Autodesk Fusion 360 part; units mm, degrees
note: some values were not read from the file. Set by a fixed rule: the direction of a hole.
(part 4 of 6)
  spline S731 degree 3 poles (-127.5181, -68.7033) (-127.2038, -68.7033) (-126.8894, -68.7033) (-126.5656, -68.7033) knots 0 0 0 0 1 1 1 1
  spline S732 degree 3 poles (-126.5656, -68.7033) (-126.5656, -71.637) (-126.5656, -74.5707) (-126.5656, -77.5933) knots 0 0 0 0 1 1 1 1
  spline S733 degree 3 poles (-123.0731, -62.9883) (-123.0731, -62.7264) (-123.0731, -62.4644) (-123.0731, -62.1946) knots 0 0 0 0 1 1 1 1
  spline S734 degree 3 poles (-123.0731, -62.1946) (-122.7784, -62.0963) (-122.7784, -62.0963) (-122.4778, -61.9961) knots 0 0 0 0 1 1 1 1
  spline S735 degree 3 poles (-122.4778, -61.9961) (-121.7659, -61.727) (-121.3352, -61.4302) (-120.9973, -60.7288) knots 0 0 0 0 1 1 1 1
  spline S736 degree 3 poles (-120.9973, -60.7288) (-120.8296, -60.2267) (-120.7999, -59.8033) (-120.7849, -59.2744) knots 0 0 0 0 1 1 1 1
  spline S737 degree 3 poles (-120.7849, -59.2744) (-120.7756, -58.9882) (-120.7756, -58.9882) (-120.7663, -58.6962) knots 0 0 0 0 1 1 1 1
  spline S738 degree 3 poles (-120.7663, -58.6962) (-120.7589, -58.3995) (-120.7589, -58.3995) (-120.7514, -58.0968) knots 0 0 0 0 1 1 1 1
  spline S739 degree 3 poles (-120.7514, -58.0968) (-120.7422, -57.7956) (-120.7422, -57.7956) (-120.7328, -57.4882) knots 0 0 0 0 1 1 1 1
  spline S740 degree 3 poles (-120.7328, -57.4882) (-120.7178, -56.9933) (-120.7042, -56.4983) (-120.6918, -56.0033) knots 0 0 0 0 1 1 1 1
  spline S741 degree 3 poles (-120.6918, -56.0033) (-120.4299, -56.0033) (-120.168, -56.0033) (-119.8981, -56.0033) knots 0 0 0 0 1 1 1 1
  spline S742 degree 3 poles (-119.8981, -56.0033) (-119.8981, -58.256) (-119.8981, -60.5086) (-119.8981, -62.8296) knots 0 0 0 0 1 1 1 1
  spline S743 degree 3 poles (-119.8981, -62.8296) (-120.16, -62.8296) (-120.422, -62.8296) (-120.6918, -62.8296) knots 0 0 0 0 1 1 1 1
  spline S744 degree 3 poles (-120.6918, -62.8296) (-120.7442, -62.62) (-120.7966, -62.4105) (-120.8506, -62.1946) knots 0 0 0 0 1 1 1 1
  spline S745 degree 3 poles (-120.8506, -62.1946) (-120.975, -62.2961) (-121.0994, -62.3976) (-121.2276, -62.5021) knots 0 0 0 0 1 1 1 1
  spline S746 degree 3 poles (-121.2276, -62.5021) (-121.8807, -63.0153) (-122.2467, -63.0036) (-123.0731, -62.9883) knots 0 0 0 0 1 1 1 1
  spline S747 degree 3 poles (-70.6856, -60.2896) (-71.484, -60.1833) (-72.1646, -59.8489) (-72.8901, -59.5181) knots 0 0 0 0 1 1 1 1
  spline S748 degree 3 poles (-72.8901, -59.5181) (-73.0942, -59.4262) (-73.0942, -59.4262) (-73.3024, -59.3323) knots 0 0 0 0 1 1 1 1
  spline S749 degree 3 poles (-73.3024, -59.3323) (-73.5901, -59.2025) (-73.8777, -59.0722) (-74.165, -58.9416) knots 0 0 0 0 1 1 1 1
  spline S750 degree 3 poles (-74.165, -58.9416) (-74.6001, -58.7439) (-75.0357, -58.5474) (-75.4713, -58.3511) knots 0 0 0 0 1 1 1 1
  spline S751 degree 3 poles (-75.4713, -58.3511) (-78.1374, -57.147) (-78.1374, -57.147) (-79.4168, -56.4796) knots 0 0 0 0 1 1 1 1
  spline S752 degree 3 poles (-79.4168, -56.4796) (-79.3645, -56.27) (-79.3121, -56.0605) (-79.2581, -55.8446) knots 0 0 0 0 1 1 1 1
  spline S753 degree 3 poles (-79.2581, -55.8446) (-77.9251, -56.2478) (-76.6807, -56.8221) (-75.4183, -57.4023) knots 0 0 0 0 1 1 1 1
  spline S754 degree 3 poles (-75.4183, -57.4023) (-75.1011, -57.5475) (-74.7838, -57.6925) (-74.4664, -57.8372) knots 0 0 0 0 1 1 1 1
  spline S755 degree 3 poles (-74.4664, -57.8372) (-74.2574, -57.9325) (-74.0485, -58.0282) (-73.8397, -58.124) knots 0 0 0 0 1 1 1 1
  spline S756 degree 3 poles (-73.8397, -58.124) (-73.3173, -58.3627) (-72.7932, -58.5931) (-72.2615, -58.8102) knots 0 0 0 0 1 1 1 1
  spline S757 degree 3 poles (-72.2615, -58.8102) (-72.1586, -58.8526) (-72.0557, -58.8949) (-71.9497, -58.9386) knots 0 0 0 0 1 1 1 1
  spline S758 degree 3 poles (-71.9497, -58.9386) (-71.6668, -59.0542) (-71.3829, -59.1677) (-71.099, -59.2811) knots 0 0 0 0 1 1 1 1
  spline S759 degree 3 poles (-71.099, -59.2811) (-70.6856, -59.4958) (-70.6856, -59.4958) (-70.5268, -59.9721) knots 0 0 0 0 1 1 1 1
  spline S760 degree 3 poles (-70.5268, -59.9721) (-70.5792, -60.0768) (-70.6316, -60.1816) (-70.6856, -60.2896) knots 0 0 0 0 1 1 1 1
  spline S761 degree 3 poles (-127.5181, -62.8296) (-127.8324, -62.8296) (-128.1467, -62.8296) (-128.4706, -62.8296) knots 0 0 0 0 1 1 1 1
  spline S762 degree 3 poles (-128.4706, -62.8296) (-128.4706, -60.5769) (-128.4706, -58.3242) (-128.4706, -56.0033) knots 0 0 0 0 1 1 1 1
  spline S763 degree 3 poles (-128.4706, -56.0033) (-128.1563, -56.0033) (-127.8419, -56.0033) (-127.5181, -56.0033) knots 0 0 0 0 1 1 1 1
  spline S764 degree 3 poles (-127.5181, -56.0033) (-127.5181, -58.256) (-127.5181, -60.5086) (-127.5181, -62.8296) knots 0 0 0 0 1 1 1 1
  spline S765 degree 3 poles (-54.6518, -79.9746) (-54.9693, -79.8158) (-54.9693, -79.8158) (-55.1657, -79.2275) knots 0 0 0 0 1 1 1 1
  spline S766 degree 3 poles (-55.1657, -79.2275) (-55.2393, -78.9651) (-55.3114, -78.7023) (-55.3823, -78.4392) knots 0 0 0 0 1 1 1 1
  spline S767 degree 3 poles (-55.3823, -78.4392) (-55.4206, -78.3003) (-55.459, -78.1615) (-55.4984, -78.0184) knots 0 0 0 0 1 1 1 1
  spline S768 degree 3 poles (-55.4984, -78.0184) (-55.5794, -77.7239) (-55.6597, -77.4293) (-55.7394, -77.1344) knots 0 0 0 0 1 1 1 1
  spline S769 degree 3 poles (-55.7394, -77.1344) (-55.8613, -76.6841) (-55.9857, -76.2346) (-56.1104, -75.7851) knots 0 0 0 0 1 1 1 1
  spline S770 degree 3 poles (-56.1104, -75.7851) (-56.1886, -75.499) (-56.2668, -75.2129) (-56.3448, -74.9268) knots 0 0 0 0 1 1 1 1
  spline S771 degree 3 poles (-56.3448, -74.9268) (-56.382, -74.7925) (-56.4192, -74.6582) (-56.4575, -74.5198) knots 0 0 0 0 1 1 1 1
  spline S772 degree 3 poles (-56.4575, -74.5198) (-56.6262, -73.8905) (-56.7655, -73.3303) (-56.7156, -72.6721) knots 0 0 0 0 1 1 1 1
  spline S773 degree 3 poles (-56.7156, -72.6721) (-56.506, -72.6721) (-56.2965, -72.6721) (-56.0806, -72.6721) knots 0 0 0 0 1 1 1 1
  spline S774 degree 3 poles (-56.0806, -72.6721) (-55.5478, -74.4857) (-55.0153, -76.2996) (-54.503, -78.1192) knots 0 0 0 0 1 1 1 1
  spline S775 degree 3 poles (-54.503, -78.1192) (-54.4695, -78.2365) (-54.436, -78.3538) (-54.4015, -78.4747) knots 0 0 0 0 1 1 1 1
  spline S776 degree 3 poles (-54.4015, -78.4747) (-54.2723, -78.9375) (-54.1756, -79.3328) (-54.1756, -79.8158) knots 0 0 0 0 1 1 1 1
  spline S777 degree 3 poles (-54.1756, -79.8158) (-54.3328, -79.8682) (-54.4899, -79.9206) (-54.6518, -79.9746) knots 0 0 0 0 1 1 1 1
  spline S778 degree 3 poles (-52.7468, -50.1296) (-53.0088, -50.0772) (-53.2707, -50.0248) (-53.5406, -49.9708) knots 0 0 0 0 1 1 1 1
  spline S779 degree 3 poles (-53.5406, -49.9708) (-53.2103, -48.6991) (-52.8209, -47.4547) (-52.3996, -46.2104) knots 0 0 0 0 1 1 1 1
  spline S780 degree 3 poles (-52.3996, -46.2104) (-52.3411, -46.0366) (-52.2827, -45.8627) (-52.2225, -45.6836) knots 0 0 0 0 1 1 1 1
  spline S781 degree 3 poles (-52.2225, -45.6836) (-52.0802, -45.2605) (-51.9375, -44.8374) (-51.7943, -44.4146) knots 0 0 0 0 1 1 1 1
  spline S782 degree 3 poles (-51.7943, -44.4146) (-51.5848, -44.467) (-51.3752, -44.5193) (-51.1593, -44.5733) knots 0 0 0 0 1 1 1 1
  spline S783 degree 3 poles (-51.1593, -44.5733) (-51.2516, -45.3381) (-51.4067, -46.0337) (-51.6461, -46.7654) knots 0 0 0 0 1 1 1 1
  spline S784 degree 3 poles (-51.6461, -46.7654) (-51.7421, -47.0609) (-51.7421, -47.0609) (-51.8399, -47.3623) knots 0 0 0 0 1 1 1 1
  spline S785 degree 3 poles (-51.8399, -47.3623) (-51.9074, -47.567) (-51.9749, -47.7718) (-52.0424, -47.9765) knots 0 0 0 0 1 1 1 1
  spline S786 degree 3 poles (-52.0424, -47.9765) (-52.1106, -48.1856) (-52.1787, -48.3947) (-52.2467, -48.6038) knots 0 0 0 0 1 1 1 1
  spline S787 degree 3 poles (-52.2467, -48.6038) (-52.4126, -49.1126) (-52.5793, -49.6212) (-52.7468, -50.1296) knots 0 0 0 0 1 1 1 1
  spline S788 degree 3 poles (-127.5181, -65.6871) (-127.8324, -65.6871) (-128.1467, -65.6871) (-128.4706, -65.6871) knots 0 0 0 0 1 1 1 1
  spline S789 degree 3 poles (-128.4706, -65.6871) (-128.4706, -65.2156) (-128.4706, -64.7441) (-128.4706, -64.2583) knots 0 0 0 0 1 1 1 1
  spline S790 degree 3 poles (-128.4706, -64.2583) (-128.1563, -64.2583) (-127.8419, -64.2583) (-127.5181, -64.2583) knots 0 0 0 0 1 1 1 1
  spline S791 degree 3 poles (-127.5181, -64.2583) (-127.5181, -64.7298) (-127.5181, -65.2013) (-127.5181, -65.6871) knots 0 0 0 0 1 1 1 1
  spline S792 degree 3 poles (-126.5656, -81.0858) (-126.8799, -81.0858) (-127.1942, -81.0858) (-127.5181, -81.0858) knots 0 0 0 0 1 1 1 1
  spline S793 degree 3 poles (-127.5181, -81.0858) (-127.5181, -80.6143) (-127.5181, -80.1428) (-127.5181, -79.6571) knots 0 0 0 0 1 1 1 1
  spline S794 degree 3 poles (-127.5181, -79.6571) (-127.2038, -79.6571) (-126.8894, -79.6571) (-126.5656, -79.6571) knots 0 0 0 0 1 1 1 1
  spline S795 degree 3 poles (-126.5656, -79.6571) (-126.5656, -80.1286) (-126.5656, -80.6) (-126.5656, -81.0858) knots 0 0 0 0 1 1 1 1
extrude "Extrude4" cut sketch "Sketch2" against normal blind 0.5 contours S0 S1 S2 S3 S4 S5 S6 S7 S8 S9 S10 S11 S12 S13 S14 S15 S16 S17 S18 S19 S20 S21 S22 S23 S24 S25 S26 S27 S28 S29 S30 S31 S32 S33 S34 S35 S36 S37 S38 S39 S40 S41 S42 S43 S44 S45 S46 S47 S48 S49 S50 S51 S52 S53 S54 S55 S56 S57 S58 S59 S60 S61 S62 S63 S64 S65 S66 S67 S68 S69 S70 S71 S72 S73 S74 S75 S76 S77 S78 S79 S80 S81 S82 S83 S84 S85 S86 S87 S88 S89 S90 S91 S92 S93 S94 S95 S96 S97 S98 S99 S100 S101 S102 S103 S104 S105 S106 S107 S108 S109 S110 S111 S112 S113 S114 S115 S116 S117 S118 S119 S120 S121 S122 S123 S124 S125 S126 S127 S128 S129 S130 S131 S132 S133 S134 S135 S136 S137 S138 S139 S140 S141 S142 S143 S144 S145 S146 S147 | S148 S149 S150 S151 S152 S153 S154 S155 S156 S157 S158 S159 S160 S161 S162 S163 S164 S165 S166 S167 S168 S169 S170 S171 S172 S173 S174 S175 S176 S177 S178 S179 S180 S181 S182 S183 S184 S185 S186 S187 S188 S189 S190 S191 S192 S193 S194 S195 S196 S197 S198 S199 S200 S201 S202 S203 S204 S205 S206 S207 S208 S209 S210 S211 S212 S213 S214 S215 S216 S217 S218 S219 S220 S221 S222 S223 S224 S225 S226 S227 S228 S229 S230 S231 S232 S233 S234 S235 S236 S237 S238 | S239 S240 S241 S242 S243 S244 S245 S246 S247 S248 S249 S250 S251 S252 S253 S254 S255 S256 S257 S258 S259 S260 S261 S262 S263 S264 S265 S266 S267 | S276 S277 S278 S279 S280 S281 S282 S283 S284 S285 S286 S287 S288 S289 S290 S291 S292 S293 S294 S295 S296 S297 S298 | S308 S309 S310 S311 S312 S313 S314 S315 S316 S317 S318 S319 S320 S321 S322 | S327 S328 S329 S330 S331 S332 S333 S334 S335 S336 S337 S338 S339 S340 S341 | S346 S347 S348 S349 S350 S351 S352 S353 S354 S355 S356 S357 S358 S359 S360 S361 S362 S363 S364 S365 S366 S367 S368 S369 S370 S371 S372 S373 S374 S375 S376 S377 S378 S379 S380 S381 | S382 S383 S384 S385 S386 S387 S388 | S396 S397 S398 S399 S400 S401 S402 S403 S404 S405 S406 S407 S408 S409 S410 S411 S412 S413 S414 S415 S416 S417 S418 S419 S420 S421 S422 S423 S424 | S425 S426 S427 S428 S429 S430 S431 S432 S433 S434 S435 S436 S437 S438 S439 S440 S441 S442 S443 | S444 S445 S446 S447 S448 S449 S450 S451 S452 S453 S454 S455 S456 S457 S458 S459 S460 S461 | S462 S463 S464 S465 S466 S467 S468 S469 S470 S471 S472 S473 S474 S475 S476 S477 S478 S479 | S480 S481 S482 S483 S484 S485 S486 S487 S488 S489 S490 S491 S492 S493 S494 S495 S496 S497 S498 S499 S500 S501 S502 S503 | S504 S505 S506 S507 S508 S509 S510 | S519 S520 S521 S522 S523 S524 S525 | S533 S534 S535 S536 S537 S538 S539 S540 S541 S542 S543 S544 S545 S546 S547 S548 S549 S550 S551 S552 S553 S554 S555 S556 S557 S558 | S559 S560 S561 S562 S563 S564 S565 S566 S567 S568 S569 S570 S571 S572 S573 S574 S575 S576 S577 S578 S579 S580 S581 S582 | S583 S584 S585 S586 S587 S588 S589 S590 S591 S592 S593 S594 S595 S596 S597 S598 S599 S600 S601 S602 S603 S604 S605 S606 S607 S608 | S609 S610 S611 S612 S613 S614 S615 S616 S617 S618 S619 S620 S621 S622 S623 S624 S625 S626 S627 S628 S629 S630 S631 S632 | S633 S634 S635 S636 S637 S638 S639 S640 S641 S642 S643 S644 S645 S646 S647 S648 S649 S650 S651 S652 S653 S654 S655 | S656 S657 S658 S659 | S660 S661 S662 S663 S664 S665 S666 S667 S668 S669 S670 S671 S672 S673 S674 S675 S676 | S677 S678 S679 S680 S681 S682 S683 S684 S685 S686 S687 S688 S689 S690 S691 S692 S693 S694 S695 S696 | S697 S698 S699 S700 S701 S702 S703 S704 S705 S706 S707 S708 | S709 S710 S711 S712 S713 S714 S715 S716 S717 S718 S719 S720 S721 S722 S723 S724 S725 S726 S727 S728 | S729 S730 S731 S732 | S733 S734 S735 S736 S737 S738 S739 S740 S741 S742 S743 S744 S745 S746 | S747 S748 S749 S750 S751 S752 S753 S754 S755 S756 S757 S758 S759 S760 | S761 S762 S763 S764 | S765 S766 S767 S768 S769 S770 S771 S772 S773 S774 S775 S776 S777 | S778 S779 S780 S781 S782 S783 S784 S785 S786 S787 | S788 S789 S790 S791 | S792 S793 S794 S795 bodies 1
extrude "Extrude5" add sketch "Sketch1" along normal blind 2.5 contours L3 L7 L11 L24 L28 L29 L30 L31 | L1 L26 L32 L33 L34 L35 bodies 1
fillet "Fillet1" radius 1.5 4 edges at (15, 121, 3.75) (164, 121, 3.75) (164, 15, 3.75) (15, 15, 3.75) on bodies 1
fillet "Fillet1" radius 1.5 4 edges at (184, 136, 1.25) (-5, 136, 1.25) (184, 0, 1.25) (-5, -0.1171, 1.25) on bodies 1
equation "d3 = ( ( ( 179 - 129 ) / 2 ) * 1 ) * 1 mm - 10 mm"
equation "d4 = ( ( ( 136 - 86 ) / 2 ) * 1 ) * 1 mm - 10 mm"
equation "d5 = 15 mm + 10 mm"
equation "d6 = 15 mm + 10 mm"
equation "d7 = 129 mm + 10 mm + 10 mm"
equation "d8 = 86 mm + 10 mm + 10 mm"
equation "d11 = ( 15.5 / 2 ) * 1 mm"
equation "d12 = ( 15.5 / 2 ) * 1 mm"
equation "d14 = ( 15.75 / 2 ) * 1 mm"
equation "d16 = ( 15.75 / 2 ) * 1 mm"

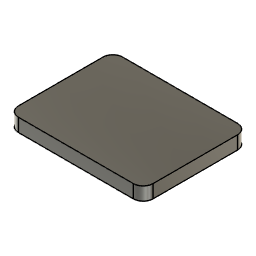
design "uv lamp"
Autodesk Fusion 360 part; units mm, degrees
sketch "Sketch1" plane through (0, 0, 0) normal (0, 0, 1) x (1, 0, 0)
  line L0 (102, -79) -> (-102, -79)
  line L1 (-102, -79) -> (-102, 79)
  line L2 (-102, 79) -> (102, 79)
  line L3 (102, 79) -> (102, -79)
  line L4 (102, -79) -> (-102, 79) construction
  line L5 (-102, -79) -> (102, 79) construction
  dimension "d1" = 204
  dimension "d2" = 158
  constraint horizontal L0
  constraint perpendicular L0 L1
  constraint parallel L0 L2
  constraint parallel L1 L3
  constraint coincident L4 origin
  constraint coincident L5 origin
  measures "d1" distance of L1.end L2.end
  measures "d2" distance of L0.end L1.end
extrude "Extrude1" add sketch "Sketch1" along normal blind 20
fillet "Fillet1" radius 15 4 edges at (102, -79, 10) (-102, -79, 10) (-102, 79, 10) (102, 79, 10)
sketch "Sketch2" plane through (0, 0, 0) normal (0, 0, -1) x (1, 0, 0)
  arc A0 (87, -79) -> (102, -64) centre (87, -64) ccw
  line L0 (102, -64) -> (102, 64)
  arc A1 (102, 64) -> (87, 79) centre (87, 64) ccw
  line L1 (87, 79) -> (-87, 79)
  arc A2 (-87, 79) -> (-102, 64) centre (-87, 64) ccw
  line L2 (-102, 64) -> (-102, -64)
  arc A3 (-102, -64) -> (-87, -79) centre (-87, -64) ccw
  line L3 (-87, -79) -> (87, -79)
  line L4 (50, -30) -> (-50, -30)
  line L5 (-50, -30) -> (-50, 30)
  line L6 (-50, 30) -> (50, 30)
  line L7 (50, 30) -> (50, -30)
  line L8 (50, -30) -> (-50, 30) construction
  line L9 (-50, -30) -> (50, 30) construction
  dimension "d7" = 100
  dimension "d8" = 60
  constraint horizontal L4
  constraint perpendicular L4 L5
  constraint parallel L4 L6
  constraint parallel L5 L7
  constraint coincident L8 origin
  constraint coincident L9 origin
  measures "d7" distance of L5.end L6.end
  measures "d8" distance of L4.end L5.end
extrude "Extrude2" add sketch "Sketch2" along normal blind 0.1 contours L4 L5 L6 L7

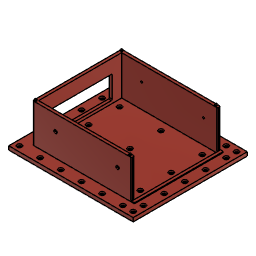
design "uv outer base"
part number: base
Autodesk Fusion 360 part; units mm, degrees
sketch "Sketch1" plane through (0, 0, 0) normal (0, 0, 1) x (1, 0, 0)
  line L0 (0, 0) -> (232, 0)
  line L1 (232, 0) -> (232, 201)
  line L2 (232, 201) -> (0, 201)
  line L3 (0, 201) -> (0, 0)
  line L4 (0, 201) -> (-7, 201)
  line L5 (0, 201) -> (-7, 201)
  line L6 (-7, 201) -> (-7, 208)
  line L7 (-7, 208) -> (0, 208)
  line L8 (0, 208) -> (0, 201)
  line L9 (232, 0) -> (239, 0)
  line L10 (239, 0) -> (239, -7)
  line L11 (239, -7) -> (232, -7)
  line L12 (232, -7) -> (232, 0)
  line L13 (-7, 208) -> (239, 208)
  line L14 (239, 208) -> (239, -7)
  line L15 (239, -7) -> (-7, -7)
  line L16 (-7, -7) -> (-7, 208)
  line L17 (232, 201) -> (232, 208)
  line L18 (239, 208) -> (239, 240.3287)
  line L19 (-21.5407, 238.3287) -> (-21.5407, 225.3287)
  line L20 (-21.5407, 225.3287) -> (-34.5407, 225.3287)
  circle A0 centre (-21.5407, -24.6713) radius 5.75
  line L21 (266.4593, -37.6713) -> (253.4593, -37.6713)
  circle A1 centre (-21.5407, 25.3287) radius 3
  line L22 (253.4593, -37.6713) -> (253.4593, -24.6713)
  circle A2 centre (-21.5407, 225.3287) radius 5.75
  line L23 (-34.5407, 238.3287) -> (-21.5407, 238.3287)
  line L24 (-34.5407, 225.3287) -> (-34.5407, 238.3287)
  line L25 (253.4593, -24.6713) -> (266.4593, -24.6713)
  circle A3 centre (28.4593, -24.6713) radius 3
  circle A4 centre (-21.5407, 225.3287) radius 3
  circle A5 centre (253.4593, 0.3287) radius 5.75
  line L26 (266.4593, -24.6713) -> (266.4593, -37.6713)
  circle A6 centre (253.4593, -24.6713) radius 5.75
  circle A7 centre (-21.5407, 25.3287) radius 5.75
  circle A8 centre (253.4593, -24.6713) radius 3
  circle A9 centre (-21.5407, 75.3287) radius 3
  circle A10 centre (253.4593, 0.3287) radius 3
  circle A11 centre (253.4593, 50.3287) radius 5.75
  circle A12 centre (253.4593, 50.3287) radius 3
  circle A13 centre (128.4593, -24.6713) radius 5.75
  circle A14 centre (78.4593, -24.6713) radius 3
  circle A15 centre (28.4593, 225.3287) radius 3
  circle A16 centre (-21.5407, -24.6713) radius 3
  circle A17 centre (228.4593, -24.6713) radius 3
  circle A18 centre (78.4593, -24.6713) radius 5.75
  circle A19 centre (253.4593, 225.3287) radius 3
  circle A20 centre (253.4593, 225.3287) radius 5.75
  circle A21 centre (-21.5407, 175.3287) radius 3
  circle A22 centre (-21.5407, 125.3287) radius 3
  circle A23 centre (-21.5407, 125.3287) radius 5.75
  circle A24 centre (28.4593, -24.6713) radius 5.75
  circle A25 centre (-21.5407, 175.3287) radius 5.75
  line L27 (232.8, 201) -> (232.8, 208)
  circle A26 centre (78.4593, 225.3287) radius 3
  circle A27 centre (178.4593, 225.3287) radius 5.75
  circle A28 centre (128.4593, 225.3287) radius 5.75
  circle A29 centre (178.4593, 225.3287) radius 3
  circle A30 centre (178.4593, -24.6713) radius 3
  circle A31 centre (128.4593, -24.6713) radius 3
  circle A32 centre (28.4593, 225.3287) radius 5.75
  circle A33 centre (228.4593, 225.3287) radius 5.75
  circle A34 centre (253.4593, 200.3287) radius 3
  line L28 (266.4593, 238.3287) -> (266.4593, -37.6713)
  circle A35 centre (128.4593, 225.3287) radius 3
  circle A36 centre (-21.5407, 75.3287) radius 5.75
  circle A37 centre (228.4593, 225.3287) radius 3
  line L29 (266.4593, -37.6713) -> (-34.5407, -37.6713)
  line L30 (-34.5407, -37.6713) -> (-34.5407, 238.3287)
  circle A38 centre (228.4593, -24.6713) radius 5.75
  circle A39 centre (78.4593, 225.3287) radius 5.75
  circle A40 centre (178.4593, -24.6713) radius 5.75
  circle A41 centre (253.4593, 200.3287) radius 5.75
  line L31 (-34.5407, 238.3287) -> (266.4593, 238.3287)
  circle A42 centre (253.4593, 100.3287) radius 5.75
  circle A43 centre (253.4593, 150.3287) radius 3
  circle A44 centre (253.4593, 100.3287) radius 3
  circle A45 centre (253.4593, 150.3287) radius 5.75
  circle A46 centre (16, 180) radius 3.375
  circle A47 centre (16, 180) radius 5.75
  circle A48 centre (116, 180) radius 3.375
  circle A49 centre (116, 180) radius 5.75
  circle A50 centre (216, 180) radius 3.375
  circle A51 centre (216, 180) radius 5.75
  circle A52 centre (16, 105) radius 3.375
  circle A53 centre (16, 105) radius 5.75
  circle A54 centre (116, 105) radius 3.375
  circle A55 centre (116, 105) radius 5.75
  circle A56 centre (216, 105) radius 3.375
  circle A57 centre (216, 105) radius 5.75
  circle A58 centre (16, 30) radius 3.375
  circle A59 centre (16, 30) radius 5.75
  circle A60 centre (116, 30) radius 3.375
  circle A61 centre (116, 30) radius 5.75
  circle A62 centre (216, 30) radius 3.375
  circle A63 centre (216, 30) radius 5.75
  point P0 (0.8, 0)
  point P1 (0.8, 0)
  point P2 (0.8, 0)
  dimension "d2" = 201
  dimension "d3" = 7
  dimension "d4" = 7
  dimension "d5" = 7
  dimension "d6" = 7
  dimension "d56" = 7
  dimension "d156" = 25
  dimension "d157" = -25
  dimension "d160" = 25
  dimension "d161" = -25
  dimension "d162" = 11.5
  dimension "d163" = 6
  dimension "d164" = 13
  dimension "d165" = 13
  dimension "d166" = 13
  dimension "d167" = 13
  dimension "d168" = 7
  dimension "d223" = 6.75
  dimension "d224" = 11.5
  dimension "d227" = 100
  dimension "d228" = -75
  constraint vertical L1
  constraint horizontal L2
  constraint vertical L3
  constraint coincident L0.start L3.end
  constraint perpendicular L3 L4
  constraint horizontal L5
  constraint vertical L6
  constraint horizontal L7
  constraint vertical L8
  constraint horizontal L13
  constraint vertical L14
  constraint vertical L16
  constraint perpendicular L13 L17
  constraint concentric A2 A4
  constraint horizontal L20
  constraint vertical L24
  constraint horizontal L23
  constraint vertical L19
  constraint coincident L19.end L20.start
  constraint horizontal L25
  constraint vertical L26
  constraint horizontal L21
  constraint vertical L22
  constraint coincident L22.end L25.start
  constraint horizontal L29
  constraint vertical L30
  constraint horizontal L31
  constraint vertical L28
  constraint concentric A46 A47
  measures "d2" distance of L0.start L2.end
  measures "d3" distance of L2.end L4.end
  measures "d4" distance of L2.end L4.end
  measures "d5" distance of L2.end L7.end
  measures "d6" distance of L0.end L9.end
  measures "d56" distance of L1.end L17.end
  measures "d162" diameter of A2
  measures "d163" diameter of A4
  measures "d164" distance of L19.end L20.end
  measures "d165" distance of L19.end L19.start
  measures "d166" distance of L22.end L25.end
  measures "d167" distance of L22.end L21.end
  measures "d168" distance of L27.end L27.start
  measures "d223" diameter of A46
  measures "d224" diameter of A47
sketch "Sketch2" plane through (0, 0, 0) normal (0, 0, 1) x (1, 0, 0)
  circle A0 centre (-22.3407, 225.3287) radius 5.75
  circle A1 centre (27.6593, 225.3287) radius 5.75
  circle A2 centre (77.6593, 225.3287) radius 5.75
  circle A3 centre (127.6593, 225.3287) radius 5.75
  circle A4 centre (177.6593, 225.3287) radius 5.75
  circle A5 centre (227.6593, 225.3287) radius 5.75
  circle A6 centre (252.6593, 225.3287) radius 5.75
  circle A7 centre (252.6593, 200.3287) radius 5.75
  circle A8 centre (-22.3407, 175.3287) radius 5.75
  circle A9 centre (252.6593, 150.3287) radius 5.75
  circle A10 centre (-22.3407, 125.3287) radius 5.75
  circle A11 centre (252.6593, 100.3287) radius 5.75
  circle A12 centre (-22.3407, 75.3287) radius 5.75
  circle A13 centre (252.6593, 50.3287) radius 5.75
  circle A14 centre (-22.3407, 25.3287) radius 5.75
  circle A15 centre (252.6593, 0.3287) radius 5.75
  circle A16 centre (-22.3407, -24.6713) radius 5.75
  circle A17 centre (27.6593, -24.6713) radius 5.75
  circle A18 centre (77.6593, -24.6713) radius 5.75
  circle A19 centre (127.6593, -24.6713) radius 5.75
  circle A20 centre (177.6593, -24.6713) radius 5.75
  circle A21 centre (227.6593, -24.6713) radius 5.75
  circle A22 centre (252.6593, -24.6713) radius 5.75
  circle A23 centre (-22.3407, 225.3287) radius 3
  circle A24 centre (27.6593, 225.3287) radius 3
  circle A25 centre (77.6593, 225.3287) radius 3
  circle A26 centre (127.6593, 225.3287) radius 3
  circle A27 centre (177.6593, 225.3287) radius 3
  circle A28 centre (227.6593, 225.3287) radius 3
  circle A29 centre (252.6593, 225.3287) radius 3
  circle A30 centre (252.6593, 200.3287) radius 3
  circle A31 centre (-22.3407, 175.3287) radius 3
  circle A32 centre (252.6593, 150.3287) radius 3
  circle A33 centre (-22.3407, 125.3287) radius 3
  circle A34 centre (252.6593, 100.3287) radius 3
  circle A35 centre (-22.3407, 75.3287) radius 3
  circle A36 centre (252.6593, 50.3287) radius 3
  circle A37 centre (-22.3407, 25.3287) radius 3
  circle A38 centre (252.6593, 0.3287) radius 3
  circle A39 centre (-22.3407, -24.6713) radius 3
  circle A40 centre (27.6593, -24.6713) radius 3
  circle A41 centre (77.6593, -24.6713) radius 3
  circle A42 centre (127.6593, -24.6713) radius 3
  circle A43 centre (177.6593, -24.6713) radius 3
  circle A44 centre (227.6593, -24.6713) radius 3
  circle A45 centre (252.6593, -24.6713) radius 3
  line L0 (-22.3407, 225.3287) -> (-35.3407, 225.3287)
  line L1 (-35.3407, 225.3287) -> (-35.3407, 238.3287)
  line L2 (-35.3407, 238.3287) -> (-22.3407, 238.3287)
  line L3 (-22.3407, 238.3287) -> (-22.3407, 225.3287)
  line L4 (252.6593, -24.6713) -> (265.6593, -24.6713)
  line L5 (265.6593, -24.6713) -> (265.6593, -37.6713)
  line L6 (265.6593, -37.6713) -> (252.6593, -37.6713)
  line L7 (252.6593, -37.6713) -> (252.6593, -24.6713)
  line L8 (265.6593, -37.6713) -> (-35.3407, -37.6713)
  line L9 (-35.3407, -37.6713) -> (-35.3407, 238.3287)
  line L10 (-35.3407, 238.3287) -> (265.6593, 238.3287)
  line L11 (265.6593, 238.3287) -> (265.6593, -37.6713)
  line L12 (232, 201) -> (232, 208)
  dimension "d8" = 11.5
  dimension "d11" = 25
  dimension "d12" = -25
  dimension "d13" = 6
  dimension "d16" = 25
  dimension "d17" = -25
  dimension "d18" = 13
  dimension "d19" = 13
  dimension "d20" = 13
  dimension "d21" = 13
  dimension "d153" = 7
  constraint concentric A0 A23
  constraint horizontal L0
  constraint vertical L1
  constraint horizontal L2
  constraint vertical L3
  constraint coincident A0.centre A23.centre
  constraint horizontal L4
  constraint vertical L5
  constraint horizontal L6
  constraint vertical L7
  constraint coincident A22.centre A45.centre
  constraint horizontal L8
  constraint vertical L9
  constraint horizontal L10
  constraint vertical L11
  measures "d8" diameter of A0
  measures "d13" diameter of A23
  measures "d18" distance of A0.centre L0.end
  measures "d19" distance of A0.centre L2.end
  measures "d20" distance of A22.centre L4.end
  measures "d21" distance of A22.centre L6.end
  measures "d153" distance of L12.start L12.end
extrude "Extrude3" add sketch "Sketch1" along normal blind 7 contours L0 L1 L2 L3 | L0 L3 L4 L5 L12 L15 L16 | L1 L9 L13 L14 L17 | L9 L10 L11 L12 L14 L15 | L2 L8 L13 L17 | L4 L5 L6 L7 L8 L13 L16 makes body 1
extrude "Extrude4" add sketch "Sketch1" along normal blind 102 contours L0 L3 L4 L5 L12 L15 L16 | L2 L8 L13 L17 | L4 L5 L6 L7 L8 L13 L16 bodies 1
sketch "Sketch4" plane through (0, 0, 102) normal (0, 0, 1) x (-1, 0, 0)
  line L0 (0, -201) -> (-232, -201)
  line L1 (-232, -201) -> (-232, -208)
  line L2 (-232, -208) -> (7, -208)
  line L3 (7, -208) -> (7, 7)
  line L4 (7, 7) -> (-232, 7)
  line L5 (-232, 0) -> (0, 0)
  line L6 (0, 0) -> (0, -201)
  line L7 (7, -208) -> (-232, -208)
  line L8 (-232, -208) -> (-232, 0)
  line L9 (-232, 0) -> (7, 0)
  line L10 (7, 0) -> (7, -208)
  line L11 (-36, -158) -> (-198, -158)
  line L12 (-198, -158) -> (-198, -43)
  line L13 (-198, -43) -> (-36, -43)
  line L14 (-36, -43) -> (-36, -158)
  line L15 (7, -208) -> (-232, -208)
  line L16 (-232, -208) -> (-232, 7)
  line L17 (-232, 7) -> (7, 7)
  line L18 (7, 7) -> (7, -208)
  line L19 (-232, 7) -> (-225, 7)
  line L20 (-225, 7) -> (-225, 3.5)
  line L21 (-225, 3.5) -> (-232, 3.5)
  line L22 (-232, 3.5) -> (-232, 7)
  line L23 (7, 7) -> (3.5, 7)
  line L24 (3.5, 7) -> (3.5, 3.5)
  line L25 (3.5, 3.5) -> (7, 3.5)
  line L26 (7, 3.5) -> (7, 7)
  line L27 (7, -208) -> (3.5, -208)
  line L28 (3.5, -208) -> (3.5, -204.5)
  line L29 (3.5, -204.5) -> (7, -204.5)
  line L30 (7, -204.5) -> (7, -208)
  line L31 (-232, -208) -> (-225, -208)
  line L32 (-225, -208) -> (-225, -204.5)
  line L33 (-225, -204.5) -> (-232, -204.5)
  line L34 (-232, -204.5) -> (-232, -208)
  line L35 (1.625, -202.625) -> (5.375, -202.625)
  line L36 (5.375, -202.625) -> (5.375, -206.375)
  line L37 (5.375, -206.375) -> (1.625, -206.375)
  line L38 (1.625, -206.375) -> (1.625, -202.625)
  line L39 (1.625, -202.625) -> (5.375, -206.375) construction
  line L40 (5.375, -202.625) -> (1.625, -206.375) construction
  line L41 (1.625, 5.375) -> (5.375, 5.375)
  line L42 (5.375, 5.375) -> (5.375, 1.625)
  line L43 (5.375, 1.625) -> (1.625, 1.625)
  line L44 (1.625, 1.625) -> (1.625, 5.375)
  line L45 (1.625, 5.375) -> (5.375, 1.625) construction
  line L46 (5.375, 5.375) -> (1.625, 1.625) construction
  line L47 (-226.875, 5.375) -> (-223.125, 5.375)
  line L48 (-223.125, 5.375) -> (-223.125, 1.625)
  line L49 (-223.125, 1.625) -> (-226.875, 1.625)
  line L50 (-226.875, 1.625) -> (-226.875, 5.375)
  line L51 (-226.875, 5.375) -> (-223.125, 1.625) construction
  line L52 (-223.125, 5.375) -> (-226.875, 1.625) construction
  line L53 (-226.875, -202.625) -> (-223.125, -202.625)
  line L54 (-223.125, -202.625) -> (-223.125, -206.375)
  line L55 (-223.125, -206.375) -> (-226.875, -206.375)
  line L56 (-226.875, -206.375) -> (-226.875, -202.625)
  line L57 (-226.875, -202.625) -> (-223.125, -206.375) construction
  line L58 (-223.125, -202.625) -> (-226.875, -206.375) construction
  line L59 (-36, -158) -> (-15.2, -158)
  line L60 (-15.2, -158) -> (-15.2, -179.35)
  line L61 (-15.2, -179.35) -> (-36, -179.35)
  line L62 (-36, -179.35) -> (-36, -158)
  line L63 (-198, -43) -> (-218.8, -43)
  line L64 (-218.8, -43) -> (-218.8, -21.65)
  line L65 (-218.8, -21.65) -> (-198, -21.65)
  line L66 (-198, -21.65) -> (-198, -43)
  line L67 (-15.2, -179.35) -> (-218.8, -179.35)
  line L68 (-218.8, -179.35) -> (-218.8, -21.65)
  line L69 (-218.8, -21.65) -> (-15.2, -21.65)
  line L70 (-15.2, -21.65) -> (-15.2, -179.35)
  line L71 (-15.2, -179.35) -> (-10.2, -179.35)
  line L72 (-10.2, -179.35) -> (-10.2, -184.35)
  line L73 (-10.2, -184.35) -> (-15.2, -184.35)
  line L74 (-15.2, -184.35) -> (-15.2, -179.35)
  line L75 (-218.8, -21.65) -> (-223.8, -21.65)
  line L76 (-223.8, -21.65) -> (-223.8, -16.65)
  line L77 (-223.8, -16.65) -> (-218.8, -16.65)
  line L78 (-218.8, -16.65) -> (-218.8, -21.65)
  line L79 (-10.2, -184.35) -> (-223.8, -184.35)
  line L80 (-223.8, -184.35) -> (-223.8, -16.65)
  line L81 (-223.8, -16.65) -> (-10.2, -16.65)
  line L82 (-10.2, -16.65) -> (-10.2, -184.35)
  line L83 (-232, 7) -> (-232, 0)
  point P0 (3.5, -204.5)
  point P1 (3.5, 3.5)
  point P2 (-225, 3.5)
  point P3 (-225, -204.5)
  dimension "d59" = 162
  dimension "d60" = 115
  dimension "d89" = 7
  dimension "d90" = 3.5
  dimension "d91" = 3.5
  dimension "d92" = 3.5
  dimension "d93" = 3.5
  dimension "d94" = 3.5
  dimension "d95" = 7
  dimension "d96" = 3.75
  dimension "d97" = 3.75
  dimension "d98" = 3.75
  dimension "d99" = 3.75
  dimension "d100" = 3.75
  dimension "d101" = 3.75
  dimension "d102" = 3.75
  dimension "d103" = 3.75
  dimension "d104" = 20.8
  dimension "d105" = 21.35
  dimension "d106" = 20.8
  dimension "d107" = 21.35
  dimension "d108" = 5
  dimension "d109" = 5
  dimension "d110" = 5
  dimension "d111" = 5
  dimension "d112" = 3.5
  constraint horizontal L7
  constraint vertical L8
  constraint horizontal L9
  constraint vertical L10
  constraint coincident L5.start L8.end
  constraint coincident L2.end L3.start
  constraint horizontal L11
  constraint vertical L12
  constraint horizontal L13
  constraint vertical L14
  constraint horizontal L15
  constraint vertical L16
  constraint horizontal L17
  constraint vertical L18
  constraint coincident L4.end L16.end
  constraint horizontal L19
  constraint vertical L20
  constraint horizontal L21
  constraint vertical L22
  constraint horizontal L23
  constraint vertical L24
  constraint horizontal L25
  constraint vertical L26
  constraint coincident L3.end L4.start
  constraint horizontal L27
  constraint vertical L28
  constraint horizontal L29
  constraint vertical L30
  constraint horizontal L31
  constraint vertical L32
  constraint horizontal L33
  constraint vertical L34
  constraint horizontal L35
  constraint perpendicular L35 L36
  constraint parallel L35 L37
  constraint parallel L36 L38
  constraint coincident L39 P0
  constraint coincident L40 P0
  constraint coincident P0 L28.end
  constraint horizontal L41
  constraint perpendicular L41 L42
  constraint parallel L41 L43
  constraint parallel L42 L44
  constraint coincident L45 P1
  constraint coincident L46 P1
  constraint coincident P1 L24.end
  constraint horizontal L47
  constraint perpendicular L47 L48
  constraint parallel L47 L49
  constraint parallel L48 L50
  constraint coincident L51 P2
  constraint coincident L52 P2
  constraint coincident P2 L20.end
  constraint horizontal L53
  constraint perpendicular L53 L54
  constraint parallel L53 L55
  constraint parallel L54 L56
  constraint coincident L57 P3
  constraint coincident L58 P3
  constraint coincident P3 L32.end
  constraint horizontal L59
  constraint vertical L60
  constraint horizontal L61
  constraint vertical L62
  constraint horizontal L63
  constraint vertical L64
  constraint horizontal L65
  constraint vertical L66
  constraint horizontal L67
  constraint vertical L68
  constraint horizontal L69
  constraint vertical L70
  constraint horizontal L71
  constraint vertical L72
  constraint horizontal L73
  constraint vertical L74
  constraint horizontal L75
  constraint vertical L76
  constraint horizontal L77
  constraint vertical L78
  constraint horizontal L79
  constraint vertical L80
  constraint horizontal L81
  constraint vertical L82
  measures "d59" distance of L11.start L11.end
  measures "d60" distance of L11.start L13.end
  measures "d89" distance of L4.end L19.end
  measures "d90" distance of L4.end L21.end
  measures "d91" distance of L3.end L23.end
  measures "d92" distance of L3.end L25.end
  measures "d93" distance of L2.end L27.end
  measures "d94" distance of L2.end L29.end
  measures "d95" distance of L1.end L31.end
  measures "d96" distance of L36.end L37.end
  measures "d97" distance of L35.end L36.end
  measures "d98" distance of L42.end L43.end
  measures "d99" distance of L41.end L42.end
  measures "d100" distance of L48.end L49.end
  measures "d101" distance of L47.end L48.end
  measures "d102" distance of L54.end L55.end
  measures "d103" distance of L53.end L54.end
  measures "d104" distance of L11.start L59.end
  measures "d105" distance of L11.start L61.end
  measures "d106" distance of L12.end L63.end
  measures "d107" distance of L12.end L65.end
  measures "d108" distance of L60.end L71.end
  measures "d109" distance of L60.end L73.end
  measures "d110" distance of L64.end L75.end
  measures "d111" distance of L64.end L77.end
  measures "d112" distance of L1.end L33.end
extrude "Extrude5" add sketch "Sketch1" along normal blind 11 contours L1 L9 L13 L14 L17 | L9 L10 L11 L12 L14 L15 bodies 1
sketch "Sketch5" plane through (0, -7, 0) normal (0, -1, 0) x (1, 0, 0)
  line L0 (-7, 0) -> (239, 0)
  line L1 (232, 11) -> (232, 102)
  line L2 (-7, 102) -> (-7, 0)
  line L3 (-7, 102) -> (15, 102)
  line L4 (0, 0) -> (0, 7)
  line L5 (15, 102) -> (232, 102)
  line L6 (232, 102) -> (232, 5.2162)
  line L7 (232, 5.2162) -> (15, 5.2162)
  line L8 (15, 5.2162) -> (15, 102)
  line L9 (0, 7) -> (48, 7)
  line L10 (48, 7) -> (48, 64.5)
  line L11 (48, 64.5) -> (0, 64.5)
  line L12 (0, 64.5) -> (0, 7)
  line L13 (48, 64.5) -> (198, 64.5)
  circle A0 centre (48, 64.5) radius 2.25
  circle A1 centre (198, 64.5) radius 2.25
  circle A2 centre (48, 64.5) radius 4
  circle A3 centre (198, 64.5) radius 4
  line L14 (232, 102) -> (-7, 102)
  line L15 (-7, 0) -> (-7, 5)
  line L16 (239, 0) -> (239, 11)
  line L17 (239, 11) -> (232, 11)
  dimension "d65" = 22
  dimension "d66" = 7
  dimension "d67" = 48
  dimension "d68" = 57.5
  dimension "d69" = 150
  dimension "d70" = 4.5
  dimension "d71" = 4.5
  dimension "d81" = 8
  dimension "d82" = 8
  constraint coincident L2.start L3.start
  constraint perpendicular L2 L3
  constraint coincident L4.start origin
  constraint perpendicular L0 L4
  constraint horizontal L5
  constraint vertical L6
  constraint horizontal L7
  constraint vertical L8
  constraint coincident L1 L6.end
  constraint horizontal L9
  constraint vertical L10
  constraint horizontal L11
  constraint vertical L12
  constraint perpendicular L10 L13
  constraint coincident L10.end L11.start
  constraint coincident L13.end A1.centre
  constraint concentric A0 A2
  constraint concentric A1 A3
  constraint coincident L0.start L2.end
  constraint coincident L2 L15.end
  constraint perpendicular L0 L15
  measures "d65" distance of L2.start L3.end
  measures "d66" distance of L4.start L4.end
  measures "d67" distance of L4.end L9.end
  measures "d68" distance of L4.end L11.end
  measures "d69" distance of L10.end L13.end
  measures "d70" diameter of A0
  measures "d71" diameter of A1
  measures "d81" diameter of A2
  measures "d82" diameter of A3
sketch "Sketch6" plane through (0, 208, 0) normal (0, 1, 0) x (-1, 0, 0)
  line L0 (-239, 0) -> (7, 0)
  line L1 (7, 0) -> (7, 102)
  line L2 (-232, 102) -> (-232, 11)
  line L3 (7, 0) -> (-15, 0)
  line L4 (-15, 0) -> (-15, 7)
  line L5 (-15, 7) -> (7, 7)
  line L6 (7, 7) -> (7, 0)
  line L7 (-15, 7) -> (-48, 7)
  line L8 (-48, 7) -> (-48, 64.5)
  line L9 (-48, 64.5) -> (-15, 64.5)
  line L10 (-15, 64.5) -> (-15, 7)
  line L11 (-48, 64.5) -> (-198, 64.5)
  circle A0 centre (-198, 64.5) radius 2.25
  circle A1 centre (-48, 64.5) radius 2.25
  circle A2 centre (-198, 64.5) radius 4
  circle A3 centre (-48, 64.5) radius 4
  line L12 (7, 102) -> (-232, 102)
  line L13 (-232, 11) -> (-239, 11)
  line L14 (-239, 11) -> (-239, 0)
  dimension "d72" = 22
  dimension "d73" = 7
  dimension "d74" = 33
  dimension "d75" = 57.5
  dimension "d76" = 150
  dimension "d77" = 4.5
  dimension "d78" = 4.5
  dimension "d83" = 8
  dimension "d84" = 8
  constraint horizontal L3
  constraint vertical L4
  constraint horizontal L5
  constraint vertical L6
  constraint coincident L0.end L1.start
  constraint horizontal L7
  constraint vertical L8
  constraint horizontal L9
  constraint vertical L10
  constraint horizontal L11
  constraint coincident L11.end A0.centre
  constraint coincident L8.end L9.start
  constraint concentric A0 A2
  constraint concentric A1 A3
  measures "d72" distance of L0.end L3.end
  measures "d73" distance of L0.end L5.end
  measures "d74" distance of L4.end L7.end
  measures "d75" distance of L4.end L9.end
  measures "d76" distance of L8.end L11.end
  measures "d77" diameter of A0
  measures "d78" diameter of A1
  measures "d83" diameter of A2
  measures "d84" diameter of A3
extrude "Extrude7" cut sketch "Sketch5" against normal blind 221 contours L11 L13 A0 | L10 L11 A0 | L10 L13 A0 | A1 bodies 1
extrude "Extrude8" cut sketch "Sketch6" against normal blind 3 contours L8 L11 A1 A3 | L8 L9 A1 A3 | L9 L11 A1 A3 | A2 bodies 1
extrude "Extrude9" cut sketch "Sketch5" against normal blind 3 contours L11 L13 A0 A2 | L10 L11 A0 A2 | L10 L13 A0 A2 | A3 bodies 1
sketch "Sketch7" plane through (0, 0, 0) normal (0, 0, 1) x (1, 0, 0)
  line L0 (632.0908, 17.9092) -> (400, 17.9092)
  line L1 (398.5, -2.5) -> (398.5, -6.5)
  line L2 (398.5, 201.5) -> (394.5, 205.5) construction
  line L3 (422.9, 178.85) -> (417.9, 178.85)
  line L4 (422.9, 183.85) -> (422.9, 178.85)
  line L5 (393, -8) -> (393, 207)
  line L6 (393, -8) -> (632, -8)
  line L7 (393, 207) -> (393, -8)
  line L8 (396.5, 207) -> (396.5, 203.5)
  line L9 (400, 17.9092) -> (400, 200)
  line L10 (393, -4.5) -> (393, -8)
  line L11 (632, 207) -> (393, 207)
  line L12 (398.5, 205.5) -> (398.5, 201.5)
  line L13 (393, 203.5) -> (393, 207)
  line L14 (632, 200) -> (632, 207)
  line L15 (394.5, 201.5) -> (394.5, 205.5)
  line L16 (396.5, -8) -> (396.5, -4.5)
  line L17 (417.9, 178.85) -> (417.9, 183.85)
  line L18 (632, -8) -> (632.0908, 17.9092)
  line L19 (394.5, -6.5) -> (398.5, -2.5) construction
  line L20 (394.5, -6.5) -> (394.5, -2.5)
  line L21 (394.5, 201.5) -> (398.5, 205.5) construction
  line L22 (400, 200) -> (632, 200)
  line L23 (396.5, -4.5) -> (393, -4.5)
  line L24 (393, 207) -> (632, 207)
  line L25 (625, 207) -> (625, 203.5)
  line L26 (627, -6.5) -> (623, -2.5) construction
  line L27 (623, -6.5) -> (623, -2.5)
  line L28 (632, 207) -> (625, 207)
  line L29 (623, -6.5) -> (627, -2.5) construction
  line L30 (623, 201.5) -> (627, 205.5) construction
  line L31 (632, 207) -> (632, -8)
  line L32 (625, -4.5) -> (632, -4.5)
  line L33 (623, -2.5) -> (627, -2.5)
  line L34 (627, -6.5) -> (623, -6.5)
  line L35 (627, -2.5) -> (627, -6.5)
  line L36 (627, 201.5) -> (623, 205.5) construction
  line L37 (632, -4.5) -> (632, -8)
  line L38 (398.5, -6.5) -> (394.5, -2.5) construction
  line L39 (393, 207) -> (396.5, 207)
  line L40 (398.5, -6.5) -> (394.5, -6.5)
  line L41 (394.5, 205.5) -> (398.5, 205.5)
  line L42 (417.9, 183.85) -> (422.9, 183.85)
  line L43 (394.5, -2.5) -> (398.5, -2.5)
  line L44 (632, -8) -> (393, -8)
  line L45 (393, -1) -> (393, 207)
  line L46 (393, -8) -> (396.5, -8)
  line L47 (632.0908, 17.9092) -> (393, -1)
  line L48 (627, 205.5) -> (627, 201.5)
  line L49 (632, 203.5) -> (632, 207)
  line L50 (631.5, 16.15) -> (626.5, 16.15)
  line L51 (632, -8) -> (625, -8)
  line L52 (625, 203.5) -> (632, 203.5)
  line L53 (625, -8) -> (625, -4.5)
  line L54 (398.5, 201.5) -> (394.5, 201.5)
  line L55 (631.5, 21.15) -> (631.5, 16.15)
  line L56 (632, 207) -> (632.0908, 17.9092)
  line L57 (393, 207) -> (632, 207)
  line L58 (623, 201.5) -> (623, 205.5)
  line L59 (623, 205.5) -> (627, 205.5)
  line L60 (627, 201.5) -> (623, 201.5)
  line L61 (396.5, 203.5) -> (393, 203.5)
  line L62 (627, 178.85) -> (632, 178.85)
  line L63 (632, 178.85) -> (632, 183.85)
  line L64 (632, 183.85) -> (627, 183.85)
  line L65 (627, 183.85) -> (627, 178.85)
  line L66 (417.9, 183.85) -> (632, 183.85)
  line L67 (632, 183.85) -> (632, 15.15)
  line L68 (632, 15.15) -> (417.9, 15.15)
  line L69 (417.9, 15.15) -> (417.9, 183.85)
  line L70 (417.9, 15.15) -> (422.9, 15.15)
  line L71 (422.9, 15.15) -> (422.9, 20.15)
  line L72 (422.9, 20.15) -> (417.9, 20.15)
  line L73 (417.9, 20.15) -> (417.9, 15.15)
  line L74 (632, 15.15) -> (627, 15.15)
  line L75 (627, 15.15) -> (627, 20.15)
  line L76 (627, 20.15) -> (632, 20.15)
  line L77 (632, 20.15) -> (632, 15.15)
  line L78 (627, 20.15) -> (422.9, 20.15)
  line L79 (422.9, 20.15) -> (422.9, 178.85)
  line L80 (422.9, 178.85) -> (627, 178.85)
  line L81 (627, 178.85) -> (627, 20.15)
  line L82 (422.9, 178.85) -> (447.9, 178.85)
  line L83 (447.9, 178.85) -> (447.9, 155.85)
  line L84 (447.9, 155.85) -> (422.9, 155.85)
  line L85 (422.9, 155.85) -> (422.9, 178.85)
  line L86 (627, 20.15) -> (602, 20.15)
  line L87 (602, 20.15) -> (602, 43.15)
  line L88 (602, 43.15) -> (627, 43.15)
  line L89 (627, 43.15) -> (627, 20.15)
  line L90 (447.9, 155.85) -> (602, 155.85)
  line L91 (602, 155.85) -> (602, 43.15)
  line L92 (602, 43.15) -> (447.9, 43.15)
  line L93 (447.9, 43.15) -> (447.9, 155.85)
  point P0 (396.5, 203.5)
  point P1 (625, -4.5)
  point P2 (625, 203.5)
  point P3 (400, -1)
  point P4 (396.5, -4.5)
  dimension "d115" = 7
  dimension "d116" = 3.5
  dimension "d117" = 3.5
  dimension "d118" = 3.5
  dimension "d119" = 3.5
  dimension "d120" = 3.5
  dimension "d121" = 7
  dimension "d122" = 4
  dimension "d123" = 4
  dimension "d124" = 4
  dimension "d125" = 4
  dimension "d126" = 4
  dimension "d127" = 4
  dimension "d128" = 4
  dimension "d129" = 4
  dimension "d134" = 5
  dimension "d135" = 5
  dimension "d138" = 3.5
  dimension "d147" = 204.1
  dimension "d188" = 5
  dimension "d189" = 5
  dimension "d190" = 168.7
  dimension "d191" = 5
  dimension "d192" = 5
  dimension "d193" = 5
  dimension "d194" = 5
  dimension "d195" = 25
  dimension "d196" = 23
  dimension "d197" = 25
  dimension "d198" = 23
  constraint coincident L0.start L18.end
  constraint coincident L5.end L7.start
  constraint coincident L6.end L18.start
  constraint coincident L5.start L6.start
  constraint perpendicular L15 L54
  constraint parallel L41 L54
  constraint parallel L12 L15
  constraint coincident P0 L2
  constraint coincident P0 L21
  constraint coincident P0 L8.end
  constraint perpendicular L20 L40
  constraint parallel L40 L43
  constraint parallel L1 L20
  constraint coincident P4 L38
  constraint coincident P4 L19
  constraint coincident P4 L16.end
  constraint perpendicular L27 L34
  constraint parallel L33 L34
  constraint parallel L27 L35
  constraint coincident P1 L26
  constraint coincident P1 L29
  constraint coincident P1 L32.start
  constraint perpendicular L58 L60
  constraint parallel L59 L60
  constraint parallel L48 L58
  constraint coincident P2 L36
  constraint coincident P2 L30
  constraint coincident P2 L25.end
  constraint horizontal L62
  constraint vertical L63
  constraint horizontal L64
  constraint vertical L65
  constraint horizontal L66
  constraint vertical L67
  constraint horizontal L68
  constraint vertical L69
  constraint horizontal L70
  constraint vertical L71
  constraint horizontal L72
  constraint vertical L73
  constraint horizontal L74
  constraint vertical L75
  constraint horizontal L76
  constraint vertical L77
  constraint horizontal L78
  constraint vertical L79
  constraint horizontal L80
  constraint vertical L81
  constraint horizontal L82
  constraint vertical L83
  constraint horizontal L84
  constraint vertical L85
  constraint horizontal L86
  constraint vertical L87
  constraint horizontal L88
  constraint vertical L89
  constraint horizontal L90
  constraint vertical L91
  constraint horizontal L92
  constraint vertical L93
  measures "d115" distance of L51.end L6.end
  measures "d116" distance of L32.end L6.end
  measures "d117" distance of L5.start L16.start
  measures "d118" distance of L5.start L10.start
  measures "d119" distance of L5.end L8.start
  measures "d120" distance of L5.end L13.start
  measures "d121" distance of L25.start L11.start
  measures "d122" distance of L2.end L12.start
  measures "d123" distance of L2.end L15.start
  measures "d124" distance of L1.start L20.end
  measures "d125" distance of L19.start L20.end
  measures "d126" distance of L26.end L29.end
  measures "d127" distance of L27.start L26.end
  measures "d128" distance of L36.end L30.end
  measures "d129" distance of L36.end L30.start
  measures "d134" distance of L3.start L3.end
  measures "d135" distance of L4.start L3.start
  measures "d138" distance of L49.start L11.start
  measures "d147" distance of L62.start L3.start
  measures "d188" distance of L62.start L62.end
  measures "d189" distance of L62.start L64.end
  measures "d190" distance of L17.end L68.end
  measures "d191" distance of L68.end L70.end
  measures "d192" distance of L68.end L72.end
  measures "d193" distance of L67.end L74.end
  measures "d194" distance of L67.end L76.end
  measures "d195" distance of L3.start L82.end
  measures "d196" distance of L3.start L84.end
  measures "d197" distance of L75.end L86.end
  measures "d198" distance of L75.end L88.end
extrude "Extrude10" add sketch "Sketch7" along normal blind 7 separate body contours L0 L31 L47 L55 L67 L77 | L0 L31 L55 L67 L76 L77 | L6 L31 L32 L34 L35 L37 L44 L51 L53 | L31 L47 L50 L55 L67 L68 L74 L75 L77 | L11 L14 L24 L25 L28 L31 L48 L49 L52 L56 L57 L59 | L0 L5 L7 L8 L9 L11 L12 L14 L15 L22 L24 L25 L31 L41 L45 L47 L48 L52 L54 L57 L58 L59 L60 L61 L68 L69 L70 L73 | L0 L47 L55 L75 | L0 L55 L75 L76 | L31 L62 L67 L76 L81 L89 | L1 L5 L6 L7 L16 L20 L23 L27 L31 L32 L33 L34 L35 L40 L43 L44 L47 L53 L68 L74 | L47 L50 L55 L75 | L0 L9 L17 L22 L31 L42 L64 L66 L69 L73 | L25 L48 L52 L59 | L25 L48 L52 L58 L59 L60 | L0 L47 L68 L71 L75 | L0 L71 L75 L78 L86 | L31 L62 L63 L64 L65 L66 L67 | L5 L6 L7 L10 L16 L20 L23 L40 L44 L46 | L32 L34 L35 L53 | L27 L32 L33 L34 L35 L53 | L47 L68 L75 | L0 L68 L69 L70 L71 L73 | L0 L69 L71 L72 L73 | L78 L81 L86 L87 L88 L89 | L4 L65 L66 L80 L82 | L80 L81 L83 L88 L90 L91 | L16 L20 L23 L40 | L1 L16 L20 L23 L40 L43 | L5 L7 L8 L11 L13 L15 L24 L39 L41 L45 L57 L61 | L78 L79 L84 L87 L92 L93 | L3 L69 L72 L79 L85 | L79 L80 L82 L83 L84 L85 | L3 L4 L17 L42 L66 L69 | L8 L12 L15 L41 L54 L61 | L8 L15 L41 L61 | L90 L91 L92 L93 makes body 2
extrude "Extrude13" cut sketch "Sketch7" along normal blind 3.5 contours L25 L48 L52 L59 | L25 L48 L52 L58 L59 L60 | L32 L34 L35 L53 | L27 L32 L33 L34 L35 L53 | L16 L20 L23 L40 | L1 L16 L20 L23 L40 L43 | L8 L12 L15 L41 L54 L61 | L8 L15 L41 L61 bodies 2
extrude "Extrude14" add sketch "Sketch1" along normal blind 9 separate body contours L19 L20 L22 A2 L25 A6 L28 L29 L30 L31 | L19 L20 A2 L23 L24 L30 L31 | L21 L22 L25 L26 A6 L28 L29 makes body 3
extrude "Extrude15" add sketch "Sketch1" along normal blind 5 contours L19 L20 A2 A4 | L19 L20 A2 A4 | L22 L25 A6 A8 | L22 L25 A6 A8 | A0 | A5 | A7 | A11 | A13 | A18 | A20 | A23 | A24 | A25 | A27 | A28 | A32 | A33 | A36 | A38 | A39 | A40 | A41 | A42 | A45 bodies 3 1
sketch "Sketch9" plane through (0, 0, 9) normal (0, 0, 1) x (-1, 0, 0)
extrude "Extrude16" add sketch "Sketch7" along normal blind 14 contours L0 L31 L47 L55 L67 L77 | L0 L31 L55 L67 L76 L77 | L31 L47 L50 L55 L67 L68 L74 L75 L77 | L0 L47 L55 L75 | L0 L55 L75 L76 | L31 L62 L67 L76 L81 L89 | L47 L50 L55 L75 | L0 L47 L68 L71 L75 | L0 L71 L75 L78 L86 | L31 L62 L63 L64 L65 L66 L67 | L47 L68 L75 | L0 L68 L69 L70 L71 L73 | L0 L69 L71 L72 L73 | L4 L65 L66 L80 L82 | L3 L69 L72 L79 L85 | L3 L4 L17 L42 L66 L69 bodies 2
extrude "Extrude17" cut sketch "Sketch7" along normal blind 7 contours L90 L91 L92 L93 bodies 2
fillet "Fillet3" radius 2 2 edges at (417.9, 183.85, 10.5) (632, 183.85, 10.5) on bodies 2
fillet "Fillet3" radius 2 2 edges at (417.9, 15.15, 10.5) (632, 15.15, 10.5) on bodies 2